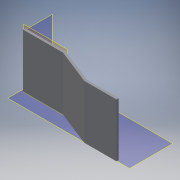
# Autodesk Inventor part: Lock1
Saved by Autodesk Inventor 2019 (Build 230136000, 136)
## iProperties
Created: 2019-11-29
Part Number: Lock1
Material: Generic
Document SubType Name: Modeling
Designer: Filip
Density: 1 g/cm^3
Appearance: Default
Author: Filip
Autodesk Inventor part; units mm, degrees
ref_plane "YZ Plane" through (0, 0, 0) normal (1, 0, 0) x (0, 1, 0)
ref_plane "XZ Plane" through (0, 0, 0) normal (0, 1, 0) x (-1, 0, 0)
ref_plane "XY Plane" through (0, 0, 0) normal (0, 0, 1) x (1, 0, 0)
ref_plane "Work Plane1" through (0, 0, 0) normal (0, 0, 1) x (1, 0, 0)
ref_plane "Work Plane2" through (-64.971, 55, -60) normal (-1, 0, 0) x (0, 0, 1)
sketch "Sketch2" plane through (-64.971, 55, -60) normal (-1, 0, 0) x (0, 0, 1)
  ellipse E0 centre (4.45, -98.8108) end of major axis (-15.5398, -98.8108) minor radius 0.0934 projected
  line L0 (5, -113) -> (60, -113) projected
  line L1 (60, 3) -> (12.1238, 3) projected
  line L2 (60, 3) -> (65, 3)
  line L3 (65, 3) -> (65, -113)
  line L4 (65, -113) -> (60, -113)
  line L5 (60, -113) -> (60, 3)
  point P0 (60, -55)
  dimension "d2" = 5
  constraints: 8 end point, 2 parallel, 1 horizontal, 1 perpendicular, 1 point on line, 1 other
  measures "d2" distance between parallel lines of L5 L3
ref_plane "Work Plane3" through (-61.971, -58, -60) normal (0, -1, 0) x (1, 0, 0)
sketch "Sketch3" plane through (-61.971, -58, -60) normal (0, -1, 0) x (1, 0, 0)
  line L0 (-3, 65) -> (-3, 60) projected
  line L1 (5, 60) -> (84, 60) projected
  line L2 (160.0104, 90) -> (84, 60) projected
  line L3 (160.0104, 90) -> (221.6846, 90) projected
  line L4 (-3, 62.5) -> (84, 62.5)
  line L5 (84, 62.5) -> (160.0104, 92.5)
  spline S0 degree 3 poles (221.6846, 90) (223.5782, 90.3311) (225.4462, 90.6526) (226.8152, 90.8725) (228.4747, 91.1391) (229.032, 91.2163) (229.4035, 91.2679) knots 0 0 0 0 0.710077 0.710077 0.710077 1.570796 1.570796 1.570796 1.570796 projected
  line L6 (160.0104, 92.5) -> (229.4035, 92.5)
  point P0 (61.971, 60)
  constraints: 6 end point, 2 horizontal, 1 midpoint, 1 parallel
sweep "Sweep1" add profiles "Sketch2" path "Sketch3" path curves L4 L5 L6 contours L2 L3 L4 L5
body "Solid1"
